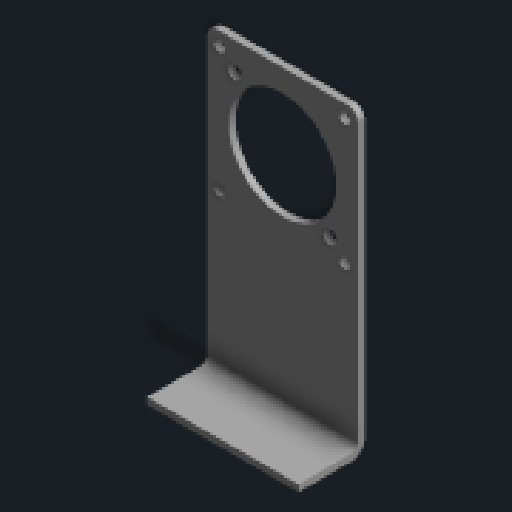
# Autodesk Inventor part: NeckStepperCover
Saved by Autodesk Inventor 2025.2 (Build 292293000, 293)
## iProperties
Created: 2025-09-16
Part Number: NeckStepperCover
Material: Generic
Document SubType Name: Sheet Metal
Designer: valer
Density: 1 g/cm^3
Sheet Metal Rule: Default
Appearance: Default
Author: valer
Autodesk Inventor part; units mm, degrees
ref_plane "YZ Plane" through (0, 0, 0) normal (1, 0, 0) x (0, 1, 0)
ref_plane "XZ Plane" through (0, 0, 0) normal (0, 1, 0) x (-1, 0, 0)
ref_plane "XY Plane" through (0, 0, 0) normal (0, 0, 1) x (1, 0, 0)
sketch "Base" plane through (0, 0, 0) normal (0, 0, 1) x (1, 0, 0)
  circle A0 centre (0, 0) radius 19.125 construction
  arc A1 (28.5, 24.5) -> (24.5, 28.5) centre (24.5, 24.5) ccw
  line L0 (24.5, 28.5) -> (-24.5, 28.5)
  arc A2 (-24.5, 28.5) -> (-28.5, 24.5) centre (-24.5, 24.5) ccw
  line L1 (-28.5, 24.5) -> (-28.5, -24.5)
  arc A3 (-28.5, -24.5) -> (-24.5, -28.5) centre (-24.5, -24.5) ccw
  line L2 (-24.5, -28.5) -> (24.5, -28.5)
  arc A4 (24.5, -28.5) -> (28.5, -24.5) centre (24.5, -24.5) ccw
  line L3 (28.5, -24.5) -> (28.5, 24.5)
  circle A5 centre (-23.57, 23.57) radius 2
  circle A6 centre (23.57, 23.57) radius 2
  circle A7 centre (-23.57, -23.57) radius 2
  circle A8 centre (23.57, -23.57) radius 2
  circle A9 centre (0, 0) radius 20.125
  circle A10 centre (-17.9605, 17.9605) radius 2.489
  circle A11 centre (17.9605, -17.9605) radius 2.489
  point P0 (0, 0)
  dimension "d0" = 1
  measures "d0" radial gap between concentric circles of A0 A9
extrude "Plate1" add sketch "Base" along normal blind 2.54
sketch "Sketch2" plane through (0, 0, 2.54) normal (0, 0, 1) x (1, 0, 0)
  line L0 (28.5, -24.5) -> (28.5, 24.5)
  line L1 (28.5, -24.5) -> (28.5, -84.5)
  line L2 (-28.5, 24.5) -> (-28.5, -24.5)
  line L3 (-28.5, -24.5) -> (-28.5, -84.5)
  line L4 (28.5, -84.5) -> (-28.5, -84.5)
  arc A0 (24.5, -28.5) -> (28.5, -24.5) centre (24.5, -24.5) ccw
  line L5 (24.5, -28.5) -> (-24.5, -28.5)
  arc A1 (-28.5, -24.5) -> (-24.5, -28.5) centre (-24.5, -24.5) ccw
  point P0 (0, 0)
  dimension "d2" = 60
  measures "d2" distance of L0.start L1.end
sheet face with bend "Face2" sketch "Sketch2" thickness 2.54 toward (0, 0, -1) bend radius 2.54 relief straight relief width 2.54 relief depth 1.27
bend "Bend1"
sketch "Sketch3" plane through (28.5, -81.96, 0) normal (0, -1, 0) x (1, 0, 0)
  line L0 (-57, 0) -> (0, 0)
  line L1 (0, 0) -> (0, 25)
  line L2 (0, 25) -> (-57, 25)
  line L3 (-57, 25) -> (-57, 0)
  constraints: 6 end point, 1 horizontal, 1 perpendicular, 1 vertical
edge flange "Flange1" height 25 angle 90 thickness 2.54 bend radius 2.54 thickness toward (0, -1, 0) relief straight relief width 2.54 relief depth 1.27 edges at (0, -84.5, 2.54) wall of the first edge with corners at (-28.5, -81.96, 0) (28.5, -81.96, 0) (28.5, -81.96, 25) (-28.5, -81.96, 25)
bend "Bend2"
corner "Corner1"
sketch "Sketch4" plane through (-28.5, -84.5, 25) normal (0, -1, 0) x (1, 0, 0)
  line L0 (0, 0) -> (57, 0) construction
  line L1 (28.5, 0) -> (28.5, -19.92) construction
  line L2 (57, -19.92) -> (0, -19.92) construction
  circle A0 centre (8, -8) radius 3
  circle A1 centre (49, -8) radius 3
  line L3 (0, -19.92) -> (0, 0) projected
  circle A2 centre (20.5, -8) radius 3
  circle A3 centre (36.5, -8) radius 3
  point P0 (28.5, -25)
  dimension "d18" = 6
  dimension "d19" = 8
  dimension "d20" = 8
  dimension "d21" = 8
  dimension "d22" = 8
  constraints: 4 centre point, 2 end point, 2 midpoint, 2 symmetric about line, 1 equal radius, 2 other
  measures "d18" diameter of A0
  measures "d19" distance from line of L0 A0.centre
  measures "d20" distance from line of L3 A0.centre
  measures "d21" distance from line of L1 A2.centre
  measures "d22" distance from line of L0 A2.centre
extrude "Cut1" cut sketch "Sketch4" against normal blind 2.54
equation "\"d22\" = d19"
equation "\"d23\" = Thickness"
equation "\"d1\" = Thickness"
equation "\"d3\" = BendRadius"
equation "\"d4\" = BendReliefWidth"
equation "\"d6\" = MinimumRemnant"
equation "\"d5\" = BendReliefDepth"
equation "\"d7\" = TransitionRadius"
equation "\"d8\" = BendReliefWidth"
equation "\"d9\" = BendReliefDepth"
equation "\"d10\" = MinimumRemnant"
equation "\"d11\" = TransitionRadius"
equation "\"d14\" = BendRadius"
equation "\"d15\" = CornerReliefSize"
equation "\"d16\" = GapSize"
equation "\"d17\" = JacobiRadiusSize"
equation "\"BendRadius\" = Thickness"
equation "\"BendReliefWidth\" = Thickness"
equation "\"BendReliefDepth\" = 0.5 * Thickness"
equation "\"CornerReliefSize\" = 4 * Thickness"
equation "\"MinimumRemnant\" = 2 * Thickness"
equation "\"TransitionRadius\" = BendRadius"
equation "\"JacobiRadiusSize\" = BendRadius"
equation "\"GapSize\" = Thickness"
equation "\"Thickness\" = 2.54"
body "Solid1"
